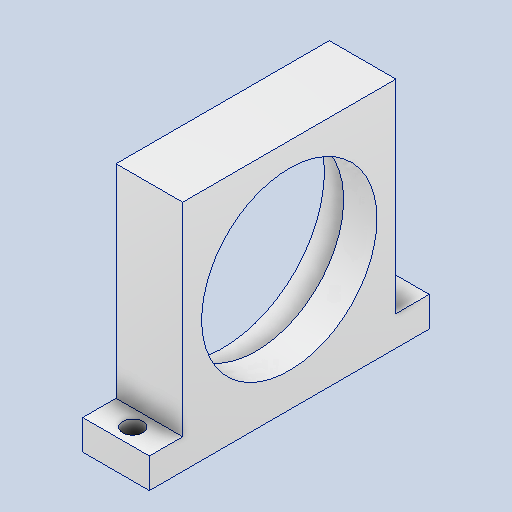
# Autodesk Inventor part: Laser holder3
Saved by Autodesk Inventor 2023 (Build 270158000, 158)
## iProperties
Created: 2023-04-11
Part Number: Laser holder3
Material: Aluminum 6061
Document SubType Name: Modeling
Designer: ASARe-DAQ-PC
Density: 2.7 g/cm^3
Appearance: Aluminum - Flat
Mass: 14.0878 g
Surface Area: 37.31 cm^2
Volume: 5.2177 cm^3
Author: ASARe-DAQ-PC
Autodesk Inventor part; units mm, degrees
ref_plane "YZ Plane" through (0, 0, 0) normal (1, 0, 0) x (0, 1, 0)
ref_plane "XZ Plane" through (0, 0, 0) normal (0, 1, 0) x (-1, 0, 0)
ref_plane "XY Plane" through (0, 0, 0) normal (0, 0, 1) x (1, 0, 0)
sketch "Sketch1" plane through (0, 0, 0) normal (1, 0, 0) x (0, 1, 0)
  line L0 (0, 0) -> (33.48, 0)
  line L1 (33.48, 0) -> (33.48, -42)
  line L2 (33.48, -42) -> (0, -42)
  line L3 (0, -42) -> (0, 0)
  point P0 (33.48, -21)
  point P1 (16.74, 0)
  dimension "d0" = 33.48
  dimension "d1" = 42
  constraints: 8 end point, 2 midpoint, 2 parallel, 1 horizontal, 1 perpendicular
  measures "d0" distance of L1.end L2.end
  measures "d1" distance between parallel lines of L0 L2
extrude "Extrusion1" add sketch "Sketch1" along normal blind 10
sketch "Sketch2" plane through (10, 0, 0) normal (1, 0, 0) x (0, 0, -1)
  line L0 (0, 33.48) -> (0, 0) projected
  line L1 (42, 33.48) -> (0, 33.48) projected
  point P0 (21, 16.74)
  point P1 (0, 16.74)
  point P2 (21, 33.48)
  constraints: 2 midpoint, 1 horizontal alignment, 1 vertical alignment
hole "Hole1" at (10, 16.74, -21) direction (-1, 0, 0) diameter 26.289 depth 66.675 tip angle 118
sketch "Sketch3" plane through (0, 0, 0) normal (0, 0, 1) x (1, 0, 0)
  line L0 (0, 0) -> (0, 33.48) projected
  line L1 (0, 33.48) -> (10, 33.48) projected
  line L2 (0, 3) -> (10, 3)
  line L3 (10, 3) -> (10, 33.48)
  line L4 (10, 33.48) -> (0, 33.48)
  line L5 (0, 33.48) -> (0, 3)
  line L6 (0, 0) -> (10, 0) projected
  dimension "d12" = 3
  constraints: 8 end point, 2 parallel, 1 horizontal, 1 perpendicular, 1 point on line
  measures "d12" distance between parallel lines of L6 L2
extrude "Extrusion2" cut sketch "Sketch3" against normal blind 5
sketch "Sketch6" plane through (0, 0, -42) normal (0, -1, 0) x (1, 0, 0)
  line L0 (0, 42) -> (0, 0) projected
  line L1 (0, 0) -> (10, 0) projected
  line L2 (0, 42) -> (10, 42)
  line L3 (10, 42) -> (10, 0)
  line L4 (10, 0) -> (0, 0)
  line L5 (0, 0) -> (0, 42)
  constraints: 8 end point, 2 parallel, 1 horizontal, 1 perpendicular
extrude "Extrusion3" add sketch "Sketch6" along normal blind 1.5
ref_plane "Work Plane1" through (0, 0, -21) normal (0, 0, 1) x (1, 0, 0)
sketch "Sketch4" plane through (0, 3, 0) normal (0, 1, 0) x (1, 0, 0)
  line L0 (10, 5) -> (10, 0) projected
  line L1 (10, 0) -> (0, 0) projected
  point P0 (5, 2.5)
  point P1 (10, 2.5)
  point P2 (5, 0)
  constraints: 2 midpoint, 1 horizontal alignment, 1 vertical alignment
hole "Hole2" at (5, 3, -2.5) direction (0, -1, 0) diameter 3 end through all
mirror "Mirror1" about plane through (0, 0, -21) normal (0, 0, 1) of "Hole2", "Extrusion2"
sketch "Sketch5" plane through (0, 0, 0) normal (-1, 0, 0) x (0, 0, 1)
  circle A0 centre (-21, 16.74) radius 13.1445 projected
  point P0 (0, 0)
  constraints: 1 coincident
hole "Hole3" at (0, 16.74, -21) direction (1, 0, 0) diameter 30.48 depth 5
body "Solid1"
